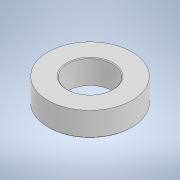
# Autodesk Inventor part: Wheel Washer
Saved by Autodesk Inventor 2022.1 (Build 261234020, 234B)
## iProperties
Created: 2023-10-18
Part Number: Wheel Washer
Material: Generic
Document SubType Name: Modeling
Designer: luke.macenski3281
Density: 1 g/cm^3
Appearance: Default
Author: luke.macenski3281
Autodesk Inventor part; units mm, degrees
ref_plane "YZ Plane" through (0, 0, 0) normal (1, 0, 0) x (0, 1, 0)
ref_plane "XZ Plane" through (0, 0, 0) normal (0, 1, 0) x (-1, 0, 0)
ref_plane "XY Plane" through (0, 0, 0) normal (0, 0, 1) x (1, 0, 0)
sketch "Sketch1" plane through (0, 0, 0) normal (0, 1, 0) x (-1, 0, 0)
  point P0 (0, 0)
sketch "Sketch2" plane through (0, 0, 0) normal (0, 1, 0) x (-1, 0, 0)
  circle A0 centre (0, 0) radius 17.78
  circle A1 centre (0, 0) radius 9.525
  dimension "d0" = 35.56
  dimension "d1" = 19.05
  constraints: 2 centre point, 2 coincident
  measures "d0" diameter of A0
  measures "d1" diameter of A1
extrude "Extrusion1" add sketch "Sketch2" along normal blind 10.16
chamfer "Chamfer1" distance 0.3175 angle 45 2 edges at (9.525, 10.16, 0) (17.78, 0, 0)
body "Solid1"
